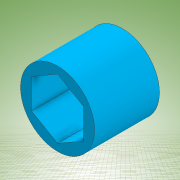
# Autodesk Inventor part: AcopleRod
Saved by Autodesk Inventor 2022 (Build 260153000, 153)
## iProperties
Created: 2022-03-09
Part Number: AcopleRod
Material: Genérico
Document SubType Name: Modeling
Designer: Marco
Density: 1 g/cm^3
Appearance: Valor por defecto
Author: Marco
Autodesk Inventor part; units mm, degrees
ref_plane "YZ Plane" through (0, 0, 0) normal (1, 0, 0) x (0, 1, 0)
ref_plane "XZ Plane" through (0, 0, 0) normal (0, 1, 0) x (-1, 0, 0)
ref_plane "XY Plane" through (0, 0, 0) normal (0, 0, 1) x (1, 0, 0)
sketch "Boceto1" plane through (0, 0, 0) normal (0, 0, 1) x (1, 0, 0)
  circle A0 centre (0, 0) radius 4
  line L0 (0, 3.2332) -> (2.8, 1.6166)
  line L1 (2.8, 1.6166) -> (2.8, -1.6166)
  line L2 (2.8, -1.6166) -> (0, -3.2332)
  line L3 (0, -3.2332) -> (-2.8, -1.6166)
  line L4 (-2.8, -1.6166) -> (-2.8, 1.6166)
  line L5 (-2.8, 1.6166) -> (0, 3.2332)
  line L6 (0, -3.2332) -> (0, -4)
  point P0 (2.8, 0)
  dimension "d0" = 8
  dimension "d1" = 5.6
  constraints: 14 end point, 2 coincident, 1 horizontal alignment, 1 midpoint, 1 vertical, 1 vertical alignment, 15 other
  measures "d1" distance of L1.end L3.end
extrude "Extrusión1" add sketch "Boceto1" along normal blind 7
